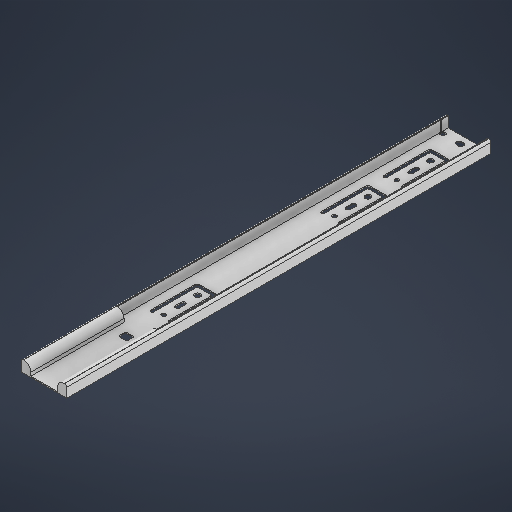
# Autodesk Inventor part: 1 часть направляшки
Saved by Autodesk Inventor 2025 (Build 290162000, 162)
## iProperties
Created: 2024-11-23
Part Number: 1 часть направляшки
Material: Типовые
Document SubType Name: Modeling
Designer: Phantom
Density: 1 g/cm^3
Appearance: По умолчанию
Author: Phantom
Autodesk Inventor part; units mm, degrees
ref_plane "YZ Plane" through (0, 0, 0) normal (1, 0, 0) x (0, 1, 0)
ref_plane "XZ Plane" through (0, 0, 0) normal (0, 1, 0) x (-1, 0, 0)
ref_plane "XY Plane" through (0, 0, 0) normal (0, 0, 1) x (1, 0, 0)
sketch "Эскиз1" plane through (0, 0, 0) normal (0, 0, 1) x (1, 0, 0)
  line L0 (0, 0) -> (-43, 0)
  line L1 (-43, 0) -> (-43, 11)
  line L2 (0, 0) -> (0, 11)
  line L3 (0, 11) -> (-3, 11)
  line L4 (-43, 11) -> (-40, 11)
  line L5 (-40, 11) -> (-40, 1)
  line L6 (-40, 1) -> (-3, 1)
  line L7 (-3, 1) -> (-3, 11)
  dimension "d0" = 43
  dimension "d1" = 11
  dimension "d2" = 11
  dimension "d3" = 3
  dimension "d4" = 10
  constraints: 16 end point, 5 perpendicular, 2 horizontal, 1 vertical
  measures "d0" distance of L0.start L0.end
  measures "d1" distance of L0.end L1.end
  measures "d2" distance of L0.start L2.end
  measures "d3" distance of L2.end L3.end
  measures "d4" distance of L4.end L5.end
extrude "Выдавливание1" add sketch "Эскиз1" along normal blind 400
sketch "Эскиз2" plane through (0, 0, 400) normal (0, 0, 1) x (1, 0, 0)
  line L0 (-40, 11) -> (-43, 11) projected
  line L1 (-43, 0) -> (0, 0) projected
  line L2 (-43, 11) -> (-34, 11)
  line L3 (-34, 11) -> (-34, 0)
  line L4 (-34, 0) -> (-43, 0)
  line L5 (-43, 0) -> (-43, 11)
  line L6 (0, 11) -> (-9, 11)
  line L7 (-9, 11) -> (-9, 0)
  line L8 (-9, 0) -> (0, 0)
  line L9 (0, 0) -> (0, 11)
  dimension "d7" = 9
  dimension "d8" = 9
  constraints: 16 end point, 4 parallel, 3 point on line, 2 horizontal, 2 perpendicular
  measures "d7" distance of L3.end L4.end
  measures "d8" distance of L8.end L7.end
extrude "Выдавливание2" add sketch "Эскиз2" against normal blind 88
fillet "Сопряжение1" radius 6.75 2 edges at (-9, 11, 356) (-34, 11, 356)
fillet "Сопряжение2" radius 2 2 edges at (-43, 11, 200) (0, 11, 200)
sketch "Эскиз3" plane through (-43, 0, 0) normal (0, -1, 0) x (1, 0, 0)
  line L0 (0, 400) -> (43, 400) projected
  line L1 (0, 0) -> (0, 400) projected
  line L2 (0, 0) -> (43, 0) projected
  line L3 (43, 0) -> (43, 400) projected
  line L4 (21.5, 400) -> (21.5, -41)
  line L5 (21.5, 400) -> (21.5, 322.5)
  line L6 (17.5, 319) -> (25.5, 319)
  line L7 (25.5, 319) -> (25.5, 326)
  line L8 (25.5, 326) -> (17.5, 326)
  line L9 (17.5, 326) -> (17.5, 319)
  line L10 (17.5, 319) -> (25.5, 326) construction
  line L11 (25.5, 319) -> (17.5, 326) construction
  line L12 (21.5, 319) -> (21.5, 287)
  circle A0 centre (21.5, 287) radius 2
  line L13 (21.5, 285) -> (21.5, 276)
  line L14 (21.5, 276) -> (21.5, 266.5) construction
  line L15 (19.5, 274) -> (19.5, 268.5)
  line L16 (23.5, 268.5) -> (23.5, 274)
  arc A1 (23.5, 274) -> (19.5, 274) centre (21.5, 274) ccw
  arc A2 (19.5, 268.5) -> (23.5, 268.5) centre (21.5, 268.5) ccw
  line L17 (21.5, 266.5) -> (21.5, 255.25)
  circle A3 centre (21.5, 255.25) radius 2.75
  line L18 (21.5, 400) -> (28.5, 400)
  line L19 (21.5, 400) -> (14.5, 400)
  line L20 (14.5, 400) -> (14.5, -41)
  line L21 (28.5, 400) -> (28.5, -41)
  line L22 (31.5, 400) -> (31.5, -41)
  line L23 (11.5, 400) -> (11.5, -41)
  line L24 (30, 291) -> (30, 247) construction
  line L25 (28.5, 289.5) -> (28.5, 248.5)
  line L26 (31.5, 248) -> (31.5, 289.5)
  arc A4 (31.5, 289.5) -> (28.5, 289.5) centre (30, 289.5) ccw
  line L27 (13, 291) -> (13, 245.5) construction
  line L28 (11.5, 289.5) -> (11.5, 248)
  line L29 (14.5, 248.5) -> (14.5, 289.5)
  arc A5 (14.5, 289.5) -> (11.5, 289.5) centre (13, 289.5) ccw
  line L30 (30, 247) -> (13, 247) construction
  line L31 (28.5, 248.5) -> (14.5, 248.5)
  line L32 (14.5, 245.5) -> (28.5, 245.5)
  arc A6 (28.5, 245.5) -> (31.5, 248.5) centre (28.75, 248.25) ccw
  arc A7 (11.5, 248.5) -> (14.5, 245.5) centre (14.25, 248.25) ccw
  circle A8 centre (21.5, 67) radius 2
  line L33 (21.5, 65) -> (21.5, 56)
  line L34 (21.5, 56) -> (21.5, 46.5) construction
  line L35 (19.5, 54) -> (19.5, 48.5)
  line L36 (23.5, 48.5) -> (23.5, 54)
  arc A9 (23.5, 54) -> (19.5, 54) centre (21.5, 54) ccw
  arc A10 (19.5, 48.5) -> (23.5, 48.5) centre (21.5, 48.5) ccw
  line L37 (21.5, 46.5) -> (21.5, 35.25)
  circle A11 centre (21.5, 35.25) radius 2.75
  line L38 (30, 71) -> (30, 27) construction
  line L39 (28.5, 69.5) -> (28.5, 28.5)
  line L40 (31.5, 28) -> (31.5, 69.5)
  arc A12 (31.5, 69.5) -> (28.5, 69.5) centre (30, 69.5) ccw
  line L41 (13, 71) -> (13, 25.5) construction
  line L42 (11.5, 69.5) -> (11.5, 28)
  line L43 (14.5, 28.5) -> (14.5, 69.5)
  arc A13 (14.5, 69.5) -> (11.5, 69.5) centre (13, 69.5) ccw
  line L44 (30, 27) -> (13, 27) construction
  line L45 (28.5, 28.5) -> (14.5, 28.5)
  line L46 (14.5, 25.5) -> (28.5, 25.5)
  arc A14 (28.5, 25.5) -> (31.5, 28.5) centre (28.75, 28.25) ccw
  arc A15 (11.5, 28.5) -> (14.5, 25.5) centre (14.25, 28.25) ccw
  circle A16 centre (21.5, 126) radius 2
  line L47 (21.5, 124) -> (21.5, 115)
  arc A17 (23.5, 113) -> (19.5, 113) centre (21.5, 113) ccw
  line L48 (23.5, 107.5) -> (23.5, 113)
  line L49 (21.5, 115) -> (21.5, 105.5) construction
  arc A18 (19.5, 107.5) -> (23.5, 107.5) centre (21.5, 107.5) ccw
  line L50 (21.5, 105.5) -> (21.5, 94.25)
  line L51 (14.5, 87.5) -> (14.5, 128.5)
  line L52 (28.5, 128.5) -> (28.5, 87.5)
  line L53 (11.5, 128.5) -> (11.5, 87)
  line L54 (31.5, 87) -> (31.5, 128.5)
  line L55 (13, 130) -> (13, 84.5) construction
  line L56 (30, 130) -> (30, 86) construction
  arc A19 (31.5, 128.5) -> (28.5, 128.5) centre (30, 128.5) ccw
  arc A20 (14.5, 128.5) -> (11.5, 128.5) centre (13, 128.5) ccw
  circle A21 centre (21.5, 94.25) radius 2.75
  line L57 (19.5, 113) -> (19.5, 107.5)
  arc A22 (28.5, 84.5) -> (31.5, 87.5) centre (28.75, 87.25) ccw
  line L58 (30, 86) -> (13, 86) construction
  line L59 (14.5, 84.5) -> (28.5, 84.5)
  arc A23 (11.5, 87.5) -> (14.5, 84.5) centre (14.25, 87.25) ccw
  line L60 (28.5, 87.5) -> (14.5, 87.5)
  line L61 (43, 7.5) -> (0, 7.5)
  line L62 (25, 7.5) -> (18, 7.5) construction
  line L63 (22.5, 10) -> (20.5, 10)
  line L64 (20.5, 5) -> (22.5, 5)
  arc A24 (22.5, 5) -> (22.5, 10) centre (22.5, 7.5) ccw
  arc A25 (20.5, 10) -> (20.5, 5) centre (20.5, 7.5) ccw
  line L65 (40.0262, 5.5287) -> (35.5266, 5.4716)
  line L66 (35.5266, 5.4716) -> (35.4758, 9.4713)
  line L67 (35.4758, 9.4713) -> (39.9755, 9.5284)
  line L68 (39.9755, 9.5284) -> (40.0262, 5.5287)
  line L69 (40.0262, 5.5287) -> (35.4758, 9.4713) construction
  line L70 (35.5266, 5.4716) -> (39.9755, 9.5284) construction
  line L71 (2.9738, 5.5287) -> (7.4734, 5.4716)
  line L72 (7.4734, 5.4716) -> (7.5242, 9.4713)
  line L73 (7.5242, 9.4713) -> (3.0245, 9.5284)
  line L74 (3.0245, 9.5284) -> (2.9738, 5.5287)
  line L75 (2.9738, 5.5287) -> (7.5242, 9.4713) construction
  line L76 (7.4734, 5.4716) -> (3.0245, 9.5284) construction
  point P0 (21.5, 271.25)
  point P1 (21.5, 289)
  point P2 (21.5, 252.5)
  point P3 (30, 268.25)
  point P4 (13, 268.25)
  point P5 (21.5, 247)
  point P6 (21.5, 51.25)
  point P7 (21.5, 69)
  point P8 (21.5, 32.5)
  point P9 (30, 48.25)
  point P10 (13, 48.25)
  point P11 (21.5, 27)
  point P12 (21.5, 69)
  point P13 (21.5, 128)
  point P14 (21.5, 110.25)
  point P15 (13, 107.25)
  point P16 (30, 107.25)
  point P17 (21.5, 91.5)
  point P18 (21.5, 86)
  point P19 (21.5, 128)
  point P20 (21.5, 128)
  point P21 (31.5, 128.5)
  point P22 (28.5, 128.5)
  point P23 (11.5, 87)
  point P24 (21.5, 7.5)
  point P25 (21.5, 7.5)
  point P26 (37.751, 7.5)
  dimension "d22" = 5.5
  dimension "d38" = 5.5
  dimension "d45" = 5.5
  dimension "d13" = 77.5
  dimension "d14" = 8
  dimension "d15" = 7
  dimension "d16" = 32
  dimension "d17" = 4
  dimension "d18" = 9
  dimension "d19" = 9.5
  dimension "d20" = 4
  dimension "d21" = 11.25
  dimension "d23" = 7
  dimension "d24" = 7
  dimension "d25" = 3
  dimension "d26" = 3
  dimension "d33" = 4
  dimension "d34" = 9
  dimension "d35" = 9.5
  dimension "d36" = 4
  dimension "d37" = 11.25
  dimension "d40" = 4
  dimension "d41" = 9
  dimension "d42" = 9.5
  dimension "d43" = 4
  dimension "d44" = 11.25
  dimension "d49" = 7.5
  dimension "d50" = 7
  dimension "d51" = 5
  dimension "d52" = 4.5
  dimension "d53" = 4
  dimension "d54" = 10.5
  constraints: 170 end point, 67 point on circle, 31 point on line, 28 tangent, 23 centre point, 19 parallel, 17 midpoint, 6 horizontal alignment, 4 coincident, 4 perpendicular, 3 vertical, 3 vertical alignment, 2 horizontal, 1 equal radius, 16 other
  measures "d13" distance of L5.start L5.end
  measures "d14" distance of L8.end L7.end
  measures "d15" distance of L7.end L6.end
  measures "d16" distance of L12.start L12.end
  measures "d17" diameter of A0
  measures "d18" distance of L13.start L13.end
  measures "d19" distance of L13.end L14.end
  measures "d20" diameter of A2
  measures "d21" distance of L14.end L17.end
  measures "d23" distance of L5.start L18.end
  measures "d24" distance of L5.start L19.end
  measures "d25" distance between parallel lines of L22 L21
  measures "d26" distance between parallel lines of L23 L20
  measures "d33" diameter of A8
  measures "d34" distance of L33.start L33.end
  measures "d35" distance of L33.end L34.end
  measures "d36" diameter of A10
  measures "d37" distance of L34.end L37.end
  measures "d40" diameter of A16
  measures "d41" distance of L47.start L47.end
  measures "d42" distance of L47.end L50.start
  measures "d43" diameter of A18
  measures "d44" distance of L50.start L50.end
  measures "d49" distance between parallel lines of L61 L2
  measures "d50" distance of L62.start L62.end
  measures "d51" diameter of A25
  measures "d52" distance of L65.start L65.end
  measures "d53" distance of L65.end L66.end
  measures "d54" distance from line of point (25, 7.5) L66
extrude "Выдавливание3" cut sketch "Эскиз3" against normal blind 88 contours A5 L20 A7 L23 | L74 L73 L72 L61 | L61 L72 L71 L74 | L8 L7 L6 L4 | L4 L6 L9 L8 | L31 L4 L32 L20 | A4 L22 A6 L21 | L31 L21 L32 L4 | A20 L20 A23 L23 | L23 A13 L20 A15 | A3 L4 | L4 A3 | L64 A25 L61 L4 | L4 L61 A24 L64 | L20 L45 L4 L46 | A25 L63 L4 L61 | A0 L4 | L4 A0 | L60 L4 L59 L20 | A16 L4 | L4 A16 | L4 L63 A24 L61 | L4 L45 L21 L46 | L68 L65 L66 L61 | L61 L66 L67 L68 | A19 L22 A22 L21 | L60 L21 L59 L4 | A2 L15 A1 L4 | L4 A1 L16 A2 | L21 A12 L22 A14 | A21 L4 | L4 A21 | A17 L48 A18 L4 | L4 A18 L57 A17 | A11 L4 | L4 A11 | A8 L4 | L4 A8 | A10 L35 A9 L4 | L4 A9 L36 A10
fillet "Сопряжение3" radius 1 18 edges at (-25.5, 0.5, 326) (-25.5, 0.5, 319) (-17.5, 0.5, 319) (-17.5, 0.5, 326) (-28.5, 0.5, 248.5) (-14.5, 0.5, 248.5) (-28.5, 0.5, 87.5) (-14.5, 0.5, 87.5) (-28.5, 0.5, 28.5) (-14.5, 0.5, 28.5) (-7.4734, 0.5, 5.4716) (-2.9738, 5.4805, 5.5287) (-3.0245, 0.5, 9.5284) (-7.5242, 0.5, 9.4713) (-35.5266, 0.5, 5.4716) (-40.0262, 5.4805, 5.5287) (-35.4758, 0.5, 9.4713) (-39.9755, 0.5, 9.5284)
